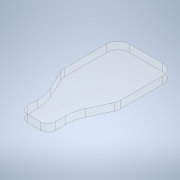
# Autodesk Inventor part: Base_plate
Saved by Autodesk Inventor 2020 (Build 240168000, 168)
## iProperties
Created: 2020-02-24
Part Number: Base_plate
Material: Acrylic, Clear
Document SubType Name: Modeling
Designer: 0x6f736f646f
Density: 1.19 g/cm^3
Appearance: Transparent - Clear
Author: 0x6f736f646f
Autodesk Inventor part; units mm, degrees
ref_plane "YZ Plane" through (0, 0, 0) normal (1, 0, 0) x (0, 1, 0)
ref_plane "XZ Plane" through (0, 0, 0) normal (0, 1, 0) x (-1, 0, 0)
ref_plane "XY Plane" through (0, 0, 0) normal (0, 0, 1) x (1, 0, 0)
sketch "Sketch1" plane through (0, 0, 0) normal (0, 1, 0) x (-1, 0, 0)
  line L0 (1.75, 15) -> (-1.75, 15)
  line L1 (-7.5, -0.6682) -> (-7.5, -12)
  line L2 (-4.5, -15) -> (4.5, -15)
  line L3 (7.5, -12) -> (7.5, -0.6682)
  line L4 (19.25, 0) -> (-19.25, 0) projected
  line L5 (0, -21.8284) -> (0, 21.6213) projected
  line L6 (3.75, 13) -> (3.75, 10.2275)
  line L7 (-3.75, 13) -> (-3.75, 10.2275)
  line L8 (4.6954, 5.9831) -> (7.2164, 0.6051)
  line L9 (-4.6954, 5.9831) -> (-7.2164, 0.6051)
  arc A0 (3.75, 10.2275) -> (4.6954, 5.9831) centre (13.75, 10.2275) ccw
  arc A1 (7.5, -0.6682) -> (7.2164, 0.6051) centre (4.5, -0.6682) ccw
  arc A2 (4.5, -15) -> (7.5, -12) centre (4.5, -12) ccw
  arc A3 (-7.5, -12) -> (-4.5, -15) centre (-4.5, -12) ccw
  arc A4 (-7.2164, 0.6051) -> (-7.5, -0.6682) centre (-4.5, -0.6682) ccw
  arc A5 (-4.6954, 5.9831) -> (-3.75, 10.2275) centre (-13.75, 10.2275) ccw
  arc A6 (3.75, 13) -> (1.75, 15) centre (1.75, 13) ccw
  arc A7 (-1.75, 15) -> (-3.75, 13) centre (-1.75, 13) ccw
  point P0 (0, 0)
  point P1 (3.75, 15)
  point P2 (-7.5, -15)
  point P3 (-7.5, 0)
  point P4 (7.5, -15)
  point P5 (0, -15)
  point P6 (3.75, 8)
  point P7 (-3.75, 8)
  point P8 (7.5, 0)
  point P9 (-3.75, 15)
  dimension "d1" = 15
  dimension "d2" = 3.75
  dimension "d3" = 3.75
  dimension "d5" = 7
  dimension "d6" = 7
  dimension "d7" = 30
  dimension "d8" = 15
  dimension "d9" = 10
  dimension "d10" = 3
  dimension "d11" = 3
  dimension "d12" = 3
  dimension "d13" = 3
  dimension "d14" = 10
  dimension "d15" = 2
  dimension "d16" = 2
  constraints: 19 point on line, 16 end point, 16 point on circle, 16 tangent, 8 centre point, 2 parallel, 2 vertical, 1 horizontal, 1 midpoint, 1 perpendicular
  measures "d1" distance of point (-7.5, -15) point (7.5, -15)
  measures "d2" distance between parallel lines of L5 L6
  measures "d3" distance between parallel lines of L5 L7
  measures "d5" distance of point (3.75, 15) point (3.75, 8)
  measures "d6" distance of point (-3.75, 15) point (-3.75, 8)
  measures "d7" distance between parallel lines of L2 L0
  measures "d8" vertical distance of point (7.5, 0) point (3.75, 15)
  measures "d9" radius of A0
  measures "d10" radius of A1
  measures "d11" radius of A2
  measures "d12" radius of A3
  measures "d13" radius of A4
  measures "d14" radius of A5
  measures "d15" radius of A6
  measures "d16" radius of A7
extrude "Extrusion1" add sketch "Sketch1" against normal blind 2
body "Solid1"
